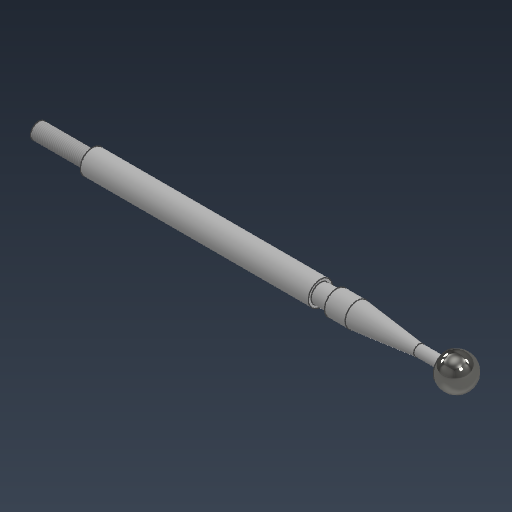
# Autodesk Inventor part: MCEN4000:T3
Saved by Autodesk Inventor 2021 (Build 250183000, 183)
## iProperties
Created: 2020-10-16
Part Number: MCEN4000:T3
Material: STEEL, AISI 1015
Document SubType Name: Modeling
Designer: Eugene Tang
Mass: 536.377 g
Surface Area: 172.187 cm^2
Volume: 68.3283 cm^3
Density: 7.85 g/cm^3
Appearance: AISI 1015
Description: TIE ROD
Screw_DIA: 12.000 mm
ScrewDEPTH: 40.000 mm
Author: Eugene Tang
Autodesk Inventor part; units mm, degrees
ref_plane "YZ Plane" through (0, 0, 0) normal (1, 0, 0) x (0, 1, 0)
ref_plane "XZ Plane" through (0, 0, 0) normal (0, 1, 0) x (-1, 0, 0)
ref_plane "XY Plane" through (0, 0, 0) normal (0, 0, 1) x (1, 0, 0)
sketch "Sketch2" plane through (0, 0, 0) normal (0, 0, 1) x (1, 0, 0)
  circle A0 centre (0, 0) radius 12.5 construction
  line L0 (-7.5, 10) -> (-7.5, 0) construction
  line L1 (-371.0321, 0) -> (76.3349, 0) construction
  line L2 (-74.125, 14.1609) -> (-74.125, -14.7732) construction
  line L3 (-28, 19.1828) -> (-28, -20.0705) construction
  line L4 (-89.5, 17.5781) -> (-89.5, -23.2799) construction
  line L5 (-101.5, 15.9734) -> (-101.5, -24.3909) construction
  line L6 (-271.5, 12.8874) -> (-271.5, -21.6752) construction
  line L7 (-7.5, 4) -> (-28, 4)
  line L8 (-28, 4) -> (-74.125, 9)
  line L9 (-89.5, 9) -> (-74.125, 9)
  line L10 (-311.5, 16.0077) -> (-311.5, -21.7095) construction
  line L11 (-89.5, 9) -> (-89.5, 7)
  line L12 (-89.5, 7) -> (-101.5, 7)
  line L13 (-101.5, 7) -> (-101.5, 9)
  line L14 (-101.5, 9) -> (-271.5, 9)
  line L15 (-311.5, 0) -> (12.5, 0)
  line L16 (-311.5, 6) -> (-271.5, 6)
  line L17 (-271.5, 9) -> (-271.5, 6)
  line L18 (-311.5, 6) -> (-311.5, 0)
  line L19 (-7.5, 4) -> (-7.5, 10)
  arc A1 (12.5, 0) -> (-7.5, 10) centre (0, 0) ccw
  dimension "d13" = 25
  dimension "d14" = 10
  dimension "d15" = 82
  dimension "d16" = 61.5
  dimension "d17" = 46.125
  dimension "d18" = 12
  dimension "d19" = 170
  dimension "ScrewDEPTH" = 40
  dimension "d21" = 4
  dimension "d22" = 9
  dimension "d23" = 7
  dimension "d24" = 6
  constraints: 38 end point, 14 point on line, 8 vertical, 4 parallel, 4 point on circle, 2 centre point, 2 perpendicular, 1 coincident, 1 collinear, 1 concentric, 1 horizontal
  measures "d13" diameter of A0
  measures "d14" distance of L0.start L0.end
  measures "d15" distance between parallel lines of L0 L4
  measures "d16" distance between parallel lines of L4 L3
  measures "d17" distance between parallel lines of L3 L2
  measures "d18" distance between parallel lines of L4 L5
  measures "d19" distance between parallel lines of L5 L6
  measures "ScrewDEPTH" distance between parallel lines of L6 L10
  measures "d21" distance between parallel lines of L15 L7
  measures "d22" distance between parallel lines of L15 L9
  measures "d23" distance between parallel lines of L15 L12
  measures "d24" distance between parallel lines of L15 L16
revolve "Revolution2" add sketch "Sketch2" angle 360 about axis through (-311.5, 0, 0) along (1, 0, 0)
thread "Thread2" size "M12x1.25" class "6g" standard "ISO Metric profile" length 40
equation "\"d13\" = BallJointBall_Dia"
equation "\"d14\" = Chord"
equation "\"d16\" = 0.75 * d15"
equation "\"d17\" = 0.75 * d16"
equation "\"d47\" = ScrewDEPTH"
equation "\"d35\" = 55deg"
equation "\"Sketch3_Pitch\" = 1.5"
equation "\"Screw_DIA\" = 2 * d24"
equation "\"d56\" = 55deg"
equation "\"Sketch6_Pitch\" = 1.25"
equation "\"BallJointBall_Dia\" = 25"
equation "\"Chord\" = 10"
body "Solid2"
